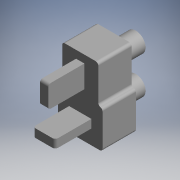
# Autodesk Inventor part: Tplug
Saved by Autodesk Inventor 2019 (Build 230136000, 136)
## iProperties
Part Number: Tplug
Material: Generic
Document SubType Name: Modeling
Designer: Jorge
Appearance: Default
Author: Jorge
## iProperties of the stored document Tplug_3DPrint.ipt
Part Number: Tplug_3DPrint
Material: Generic
Document SubType Name: Modeling
Designer: Jorge
Appearance: Default
Author: Jorge
Autodesk Inventor part; units mm, degrees
ref_plane "YZ Plane" through (0, 0, 0) normal (1, 0, 0) x (0, 1, 0)
ref_plane "XZ Plane" through (0, 0, 0) normal (0, 1, 0) x (-1, 0, 0)
ref_plane "XY Plane" through (0, 0, 0) normal (0, 0, 1) x (1, 0, 0)
sketch "Sketch1" plane through (0, 0, 0) normal (0, 0, 1) x (1, 0, 0)
  line L0 (4, 9.5) -> (4, 4) construction
  line L1 (0.75, 6.75) -> (0.75, 13.5)
  line L2 (0.75, 13.5) -> (7.25, 13.5)
  line L3 (7.25, 13.5) -> (7.25, 6.75)
  line L4 (0, 6.75) -> (0, 0)
  line L5 (0, 0) -> (8, 0)
  line L6 (8, 0) -> (8, 6.75)
  line L7 (0, 6.75) -> (0.75, 6.75)
  line L8 (7.25, 6.75) -> (8, 6.75)
  line L9 (0.75, 6.75) -> (7.25, 6.75) construction
  line L10 (4, 4) -> (4, 0) construction
  line L11 (4, 9.5) -> (4, 13.5) construction
  line L12 (3.25, 12.125) -> (4.75, 12.125)
  line L13 (4.75, 12.125) -> (4.75, 8.125)
  line L14 (4.75, 8.125) -> (3.25, 8.125)
  line L15 (3.25, 8.125) -> (3.25, 12.125)
  line L16 (2, 4.125) -> (6, 4.125)
  line L17 (6, 4.125) -> (6, 2.625)
  line L18 (6, 2.625) -> (2, 2.625)
  line L19 (2, 2.625) -> (2, 4.125)
  line L20 (4.75, 12.125) -> (4.75, 13.5) construction
  line L21 (4.75, 8.125) -> (4.75, 6.75) construction
  line L22 (6, 2.625) -> (6, 0) construction
  line L23 (6, 4.125) -> (6, 6.75) construction
  point P0 (4, 6.75)
  dimension "d2" = 5.5
  dimension "d3" = 6.5
  dimension "d4" = 8
  dimension "d5" = 13.5
  dimension "d9" = 1.5
  dimension "d10" = 4
  dimension "d11" = 4
  dimension "d12" = 1.5
  constraints: 48 end point, 8 perpendicular, 5 horizontal, 5 point on line, 4 collinear, 4 midpoint, 4 parallel, 4 vertical, 1 coincident, 4 other
  measures "d2" distance of L0.start L0.end
  measures "d3" distance of L1.end L2.end
  measures "d4" distance of L4.end L5.end
  measures "d5" distance between parallel lines of L5 L2
  measures "d9" distance of L13.end L14.end
  measures "d10" distance of L12.end L13.end
  measures "d11" distance of L17.end L18.end
  measures "d12" distance of L16.end L17.end
extrude "Extrusion2" add sketch "Sketch1" along normal blind 6
fillet "Fillet2" radius 0.5 8 edges at (7.25, 6.75, 3) (8, 6.75, 3) (0, 6.75, 3) (0.75, 6.75, 3) (0, 0, 3) (8, 0, 3) (7.25, 13.5, 3) (0.75, 13.5, 3)
extrude "Extrusion3" add sketch "Sketch1" along normal blind 12.5 contours L12 L13 L14 L15 | L16 L17 L18 L19
sketch "Sketch2" plane through (0, 0, 0) normal (0, 0, -1) x (-1, 0, 0)
  line L0 (-6, 4.125) -> (-2, 4.125) construction
  line L1 (-2, 4.125) -> (-2, 2.625) construction
  line L2 (-2, 2.625) -> (-6, 2.625) construction
  line L3 (-6, 2.625) -> (-6, 4.125) construction
  line L4 (-4.75, 12.125) -> (-3.25, 12.125) construction
  line L5 (-3.25, 12.125) -> (-3.25, 8.125) construction
  line L6 (-3.25, 8.125) -> (-4.75, 8.125) construction
  line L7 (-4.75, 8.125) -> (-4.75, 12.125) construction
  line L8 (-3.25, 8.125) -> (-3.25, 12.125) construction
  line L9 (-3.25, 12.125) -> (-4.75, 8.125) construction
  line L10 (-3.25, 12.125) -> (-4.75, 12.125) construction
  line L11 (-3.25, 8.125) -> (-4.75, 12.125) construction
  line L12 (-2, 4.125) -> (-6, 2.625) construction
  line L13 (-6, 2.625) -> (-2, 2.625) construction
  line L14 (-6, 2.625) -> (-6, 4.125) construction
  line L15 (-2, 2.625) -> (-6, 4.125) construction
  circle A0 centre (-4, 10.125) radius 1.75
  circle A1 centre (-4, 3.375) radius 1.75
  point P0 (0, 0)
  dimension "d18" = 3.5
  dimension "d19" = 3.5
  constraints: 8 end point, 2 centre point, 2 midpoint
  measures "d18" diameter of A0
  measures "d19" diameter of A1
extrude "Extrusion4" add sketch "Sketch2" along normal blind 4
fillet "Fillet3" radius 0.5 4 edges at (4, 12.125, 12.5) (4, 8.125, 12.5) (2, 3.375, 12.5) (6, 3.375, 12.5)
body "Solid2"
